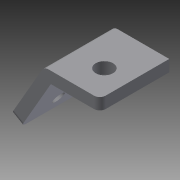
# Autodesk Inventor part: EE_adapter
Saved by Autodesk Inventor 2015 (Build 190159000, 159)
## iProperties
Created: 2014-12-11
Part Number: EE_adapter
Material: Generic
Document SubType Name: Modeling
Designer: rawrdong
Density: 1 g/cm^3
Appearance: Default
Author: rawrdong
Autodesk Inventor part; units mm, degrees
ref_plane "YZ Plane" through (0, 0, 0) normal (1, 0, 0) x (0, 1, 0)
ref_plane "XZ Plane" through (0, 0, 0) normal (0, 1, 0) x (-1, 0, 0)
ref_plane "XY Plane" through (0, 0, 0) normal (0, 0, 1) x (1, 0, 0)
sketch "Sketch1" plane through (0, 0, 0) normal (0, 1, 0) x (-1, 0, 0)
  line L0 (0.5774, -1) -> (8.6603, -15)
  line L1 (8.6603, -15) -> (6.0622, -16.5)
  line L2 (-1.1547, 0) -> (-14.4338, 0)
  line L3 (-14.4338, 0) -> (-14.4338, -3)
  line L4 (-14.4338, -3) -> (-1.7898, -3)
  line L5 (-1.7032, -3.05) -> (6.0622, -16.5)
  line L6 (0, 0) -> (-8.1844, -14.1757) construction
  arc A0 (-1.7032, -3.05) -> (-1.7898, -3) centre (-1.7898, -3.1) ccw
  arc A1 (0.5774, -1) -> (-1.1547, 0) centre (-1.1547, -2) ccw
  line L7 (-19.0526, 0) -> (13.2791, 0) projected
  point P0 (-1.7321, -3)
  dimension "d4" = 3
  dimension "d8" = 0.1
  dimension "d9" = 2
  dimension "d16" = 120
  dimension "d19" = 12.5
  dimension "d20" = 15
  constraints: 14 end point, 5 point on line, 4 point on circle, 4 tangent, 3 perpendicular, 2 centre point, 1 equal length, 1 horizontal, 1 vertical
  measures "d4" distance of L2.end L3.end
  measures "d8" radius of A0
  measures "d9" radius of A1
  measures "d16" angle of L4 L5
  measures "d19" distance from line of L2.end L0
  measures "d20" distance from line of L7 L0.end
extrude "Extrusion1" add sketch "Sketch1" along normal blind 15
sketch "Sketch2" plane through (0, 15, 0) normal (0, 1, 0) x (1, 0, 0)
  line L0 (-8.6603, 15) -> (-0.5774, 1) projected
  line L1 (1.1547, 0) -> (14.4338, 0) projected
  line L2 (14.4338, 0) -> (14.4338, 3) projected
  line L3 (14.4338, 3) -> (1.7898, 3) projected
  line L4 (1.7032, 3.05) -> (-6.0622, 16.5) projected
  line L5 (-6.0622, 16.5) -> (-8.6603, 15) projected
  line L6 (14.4338, 3) -> (-6.0622, 16.5)
  arc A0 (-0.5774, 1) -> (1.1547, 0) centre (1.1547, 2) ccw projected
  arc A1 (1.7032, 3.05) -> (1.7898, 3) centre (1.7898, 3.1) ccw projected
  point P0 (0, 0)
  constraints: 2 end point
extrude "Extrusion2" add sketch "Sketch2" along normal blind 3
sketch "Sketch3" plane through (14.4338, 0, -3) normal (0, 0, -1) x (-1, 0, 0)
  line L0 (0, 0) -> (12.644, 0) projected
  line L1 (0, 0) -> (0, 15) projected
  circle A0 centre (6.322, 7.5) radius 2.25
  line L2 (12.644, 0) -> (12.644, 15) projected
  line L3 (0, 15) -> (12.644, 15) projected
  point P0 (14.4338, 0)
  point P1 (6.322, 0)
  point P2 (0, 7.5)
  dimension "d5" = 4.5
  constraints: 2 midpoint, 1 centre point, 1 horizontal alignment, 1 vertical alignment
  measures "d5" diameter of A0
extrude "Extrusion3" cut sketch "Sketch3" against normal through all contours A0
sketch "Sketch5" plane through (-6.0622, 0, -16.5) normal (0.866, 0, -0.5) x (-0.5, 0, -0.866)
  circle A0 centre (-4.5, 7.5) radius 1.5
  line L0 (-15.5307, 0) -> (0, 0) projected
  line L1 (0, 0) -> (0, 15) projected
  line L2 (-15.5307, 15) -> (0, 15) projected
  line L3 (-15.5307, 0) -> (-15.5307, 15) projected
  point P0 (-17.3205, 0)
  point P1 (0, 7.5)
  dimension "d12" = 3
  dimension "d18" = 4.5
  constraints: 1 centre point, 1 horizontal alignment, 1 midpoint
  measures "d12" diameter of A0
  measures "d18" distance of point (0, 7.5) A0.centre
extrude "Extrusion4" cut sketch "Sketch5" against normal through all contours A0
fillet "Fillet1" radius 1.5 2 edges at (-7.3612, 0, -15.75) (14.4338, 0, -1.5)
body "Solid1"
